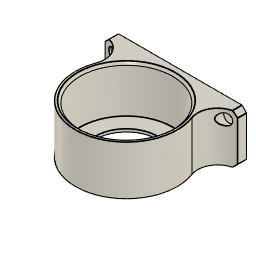
Držák IPA v1 (Autodesk Fusion 360 design; units mm, degrees)
Autodesk Fusion 360 part; units mm, degrees
note: some values were not read from the file. Set by a fixed rule: which sketch regions a step uses.
sketch "Sketch1" plane through (0, 0, 0) normal (0, 0, 1) x (1, 0, 0)
  circle A0 centre (0, 0) radius 30
  circle A1 centre (0, 0) radius 33
  line L0 (43, 33) -> (-43, 33)
  line L1 (-43, 33) -> (-43, 35)
  line L2 (-43, 35) -> (43, 35)
  line L3 (43, 35) -> (43, 33)
  line L4 (43, 33) -> (-43, 35) construction
  line L5 (-43, 33) -> (43, 35) construction
  line L6 (-33, 0) -> (-33, 33) construction
  line L7 (-43, 33) -> (-43, 29)
  arc A2 (-30.9074, 11.5642) -> (-43, 29) centre (-43, 16.0887) ccw
  line L8 (0, 2.5) -> (0, 20)
  line L9 (43, 33) -> (43, 29)
  arc A3 (43, 29) -> (30.9074, 11.5642) centre (43, 16.0887) ccw
  line L10 (-32.8634, -3) -> (-29.8496, -3)
  line L11 (29.8496, -3) -> (32.8634, -3)
  circle A4 centre (0, 0) radius 20
  point P0 (0, 34)
  dimension "d1" = 60
  dimension "d2" = 3
  dimension "d3" = 2
  dimension "d4" = 10
  dimension "d5" = 6
  dimension "d6" = 3
  dimension "d7" = 40
  constraint coincident A0.centre A1.centre
  constraint horizontal L0
  constraint perpendicular L0 L1
  constraint parallel L0 L2
  constraint parallel L1 L3
  constraint coincident L4 P0
  constraint coincident L5 P0
  constraint vertical A0.centre P0
  constraint tangent A1 L0
  constraint coincident A1 L6.start
  constraint coincident L0 L6.end
  constraint perpendicular L0 L6
  constraint tangent A1 L6
  constraint tangent A1 A2
  constraint coincident A1 A2.start
  constraint perpendicular L0 L7
  constraint vertical L0.end A2.centre
  constraint symmetric L0.end L8 L0.start
  constraint symmetric L7.end L8 L9.end
  constraint symmetric A2.start L8 A3.end
  constraint symmetric A2 L8 A3
  constraint coincident A1 L10.start
  constraint coincident A1 L11.end
  constraint horizontal L10
  constraint coincident A0 L10.end
  constraint coincident A0 L11.start
  constraint collinear L10 L11
  constraint concentric A0 A4
  measures "d1" diameter of A0
  measures "d3" distance of L0.end L1.end
  measures "d4" distance of L1 L6
  measures "d5" distance of L1.end L7.end
  measures "d6" distance of A0.centre L10
  measures "d7" diameter of A4
extrude "Extrude1" add sketch "Sketch1" against normal blind 2
extrude "Extrude2" add sketch "Sketch1" along normal blind 30 contours A0 A1 L10 L11 | A0 A1 L10 L11 | A1 L0 L7 A2 | A1 L0 L9 A3 | L0 L1 L2 L3
sketch "Sketch2" plane through (0, 35, 0) normal (0, 1, 0) x (-1, 0, 0)
  line L0 (-43, 30) -> (-43, -2)
  line L1 (-43, -2) -> (43, -2)
  line L2 (43, -2) -> (43, 30)
  line L3 (43, 30) -> (-43, 30)
  line L4 (30.9074, 30) -> (30.9074, -2)
  line L5 (-33, -2) -> (33, -2)
  line L6 (-30.9074, -2) -> (-30.9074, 30)
  line L7 (33, 30) -> (-33, 30)
  line L8 (-33, 30) -> (-33, -2) construction
  line L9 (-43, 14) -> (-33, 14) construction
  circle A0 centre (-36.5, 24) radius 1.6
  line L10 (0, 20) -> (0, 2.5)
  circle A1 centre (36.5, 24) radius 1.6
  circle A2 centre (-36.5, 24) radius 3.5
  circle A3 centre (36.5, 24) radius 3.5
  point P0 (-43, 14)
  point P1 (-36.5, 24)
  dimension "d12" = 3.2
  dimension "d14" = 7
  dimension "d39" = 6
  constraint midpoint L0 P0
  constraint coincident L7.end L8.start
  constraint coincident L5.start L8.end
  constraint coincident P0 L9.start
  constraint midpoint L8 L9.end
  constraint coincident P1 A0.centre
  constraint symmetric A0 L10 A1
  constraint symmetric L10 A2 A3
  constraint tangent L8 A2
  measures "d12" diameter of A0
  measures "d14" diameter of A2
  measures "d39" distance of L3 P1
extrude "Extrude3" cut sketch "Sketch2" against normal through all contours A0 | A1
extrude "Extrude4" cut sketch "Sketch2" against normal blind 15 from surface at -5 contours A2 | A3
chamfer "Chamfer1" distance 1.9 angle 45 2 edges at (-35.0083, 30, 24.5786) (37.9917, 30, 24.5786)
chamfer "Chamfer2" distance 3 angle 45 4 edges at (-43, 32, -2) (-43, 32, 30) (43, 32, -2) (43, 32, 30)
chamfer "Chamfer3" distance 1.5 angle 45 1 edges at (-27.9698, 10.8485, 30)
chamfer "Chamfer4" distance 0.2 angle 45 4 edges at (-33, 24.2558, 24) (40, 28.6466, 24) (-18.6465, 7.2323, 0) (-27.9698, -10.8485, 0) 9 faces at (-11.6861, 35, 6.4353) (-0.4982, 29.9814, -2) (41.4965, 32.9705, -0.5035) (43, 33, 9.6667) (31.5811, 28.6438, 30) (41.4965, 32.9705, 28.5035) (-41.4965, 32.9705, 28.5035) (-43, 31, 9.6667) (-41.4965, 32.9705, -0.5035)
named bodies: "Držák IPA"
